Autodesk Fusion 360 part; units mm, degrees
(part 2 of 3)
  line L236 (-80.5456, -102.6502) -> (-76.5456, -102.6502)
  arc A232 (-58.9345, -105.6502) -> (-61.9345, -102.6502) centre (-61.9345, -105.6502) ccw
  line L237 (-58.9345, -105.6502) -> (-58.9345, -109.6502)
  arc A233 (-61.9345, -112.6502) -> (-58.9345, -109.6502) centre (-61.9345, -109.6502) ccw
  line L238 (-61.9345, -112.6502) -> (-65.9345, -112.6502)
  arc A234 (-68.9345, -109.6502) -> (-65.9345, -112.6502) centre (-65.9345, -109.6502) ccw
  line L239 (-68.9345, -109.6502) -> (-68.9345, -105.6502)
  arc A235 (-65.9345, -102.6502) -> (-68.9345, -105.6502) centre (-65.9345, -105.6502) ccw
  line L240 (-65.9345, -102.6502) -> (-61.9345, -102.6502)
  arc A236 (-44.3234, -105.6502) -> (-47.3234, -102.6502) centre (-47.3234, -105.6502) ccw
  line L241 (-44.3234, -105.6502) -> (-44.3234, -109.6502)
  arc A237 (-47.3234, -112.6502) -> (-44.3234, -109.6502) centre (-47.3234, -109.6502) ccw
  line L242 (-47.3234, -112.6502) -> (-51.3234, -112.6502)
  arc A238 (-54.3234, -109.6502) -> (-51.3234, -112.6502) centre (-51.3234, -109.6502) ccw
  line L243 (-54.3234, -109.6502) -> (-54.3234, -105.6502)
  arc A239 (-51.3234, -102.6502) -> (-54.3234, -105.6502) centre (-51.3234, -105.6502) ccw
  line L244 (-51.3234, -102.6502) -> (-47.3234, -102.6502)
  arc A240 (-29.7123, -105.6502) -> (-32.7123, -102.6502) centre (-32.7123, -105.6502) ccw
  line L245 (-29.7123, -105.6502) -> (-29.7123, -109.6502)
  arc A241 (-32.7123, -112.6502) -> (-29.7123, -109.6502) centre (-32.7123, -109.6502) ccw
  line L246 (-32.7123, -112.6502) -> (-36.7123, -112.6502)
  arc A242 (-39.7123, -109.6502) -> (-36.7123, -112.6502) centre (-36.7123, -109.6502) ccw
  line L247 (-39.7123, -109.6502) -> (-39.7123, -105.6502)
  arc A243 (-36.7123, -102.6502) -> (-39.7123, -105.6502) centre (-36.7123, -105.6502) ccw
  line L248 (-36.7123, -102.6502) -> (-32.7123, -102.6502)
  arc A244 (-161.2123, -120.2613) -> (-164.2123, -117.2613) centre (-164.2123, -120.2613) ccw
  line L249 (-161.2123, -120.2613) -> (-161.2123, -124.2613)
  arc A245 (-164.2123, -127.2613) -> (-161.2123, -124.2613) centre (-164.2123, -124.2613) ccw
  line L250 (-164.2123, -127.2613) -> (-168.2123, -127.2613)
  arc A246 (-171.2123, -124.2613) -> (-168.2123, -127.2613) centre (-168.2123, -124.2613) ccw
  line L251 (-171.2123, -124.2613) -> (-171.2123, -120.2613)
  arc A247 (-168.2123, -117.2613) -> (-171.2123, -120.2613) centre (-168.2123, -120.2613) ccw
  line L252 (-168.2123, -117.2613) -> (-164.2123, -117.2613)
  arc A248 (-146.6011, -120.2613) -> (-149.6011, -117.2613) centre (-149.6011, -120.2613) ccw
  line L253 (-146.6011, -120.2613) -> (-146.6011, -124.2613)
  arc A249 (-149.6011, -127.2613) -> (-146.6011, -124.2613) centre (-149.6011, -124.2613) ccw
  line L254 (-149.6011, -127.2613) -> (-153.6011, -127.2613)
  arc A250 (-156.6011, -124.2613) -> (-153.6011, -127.2613) centre (-153.6011, -124.2613) ccw
  line L255 (-156.6011, -124.2613) -> (-156.6011, -120.2613)
  arc A251 (-153.6011, -117.2613) -> (-156.6011, -120.2613) centre (-153.6011, -120.2613) ccw
  line L256 (-153.6011, -117.2613) -> (-149.6011, -117.2613)
  arc A252 (-131.99, -120.2613) -> (-134.99, -117.2613) centre (-134.99, -120.2613) ccw
  line L257 (-131.99, -120.2613) -> (-131.99, -124.2613)
  arc A253 (-134.99, -127.2613) -> (-131.99, -124.2613) centre (-134.99, -124.2613) ccw
  line L258 (-134.99, -127.2613) -> (-138.99, -127.2613)
  arc A254 (-141.99, -124.2613) -> (-138.99, -127.2613) centre (-138.99, -124.2613) ccw
  line L259 (-141.99, -124.2613) -> (-141.99, -120.2613)
  arc A255 (-138.99, -117.2613) -> (-141.99, -120.2613) centre (-138.99, -120.2613) ccw
  line L260 (-138.99, -117.2613) -> (-134.99, -117.2613)
  arc A256 (-117.3789, -120.2613) -> (-120.3789, -117.2613) centre (-120.3789, -120.2613) ccw
  line L261 (-117.3789, -120.2613) -> (-117.3789, -124.2613)
  arc A257 (-120.3789, -127.2613) -> (-117.3789, -124.2613) centre (-120.3789, -124.2613) ccw
  line L262 (-120.3789, -127.2613) -> (-124.3789, -127.2613)
  arc A258 (-127.3789, -124.2613) -> (-124.3789, -127.2613) centre (-124.3789, -124.2613) ccw
  line L263 (-127.3789, -124.2613) -> (-127.3789, -120.2613)
  arc A259 (-124.3789, -117.2613) -> (-127.3789, -120.2613) centre (-124.3789, -120.2613) ccw
  line L264 (-124.3789, -117.2613) -> (-120.3789, -117.2613)
  arc A260 (-102.7678, -120.2613) -> (-105.7678, -117.2613) centre (-105.7678, -120.2613) ccw
  line L265 (-102.7678, -120.2613) -> (-102.7678, -124.2613)
  arc A261 (-105.7678, -127.2613) -> (-102.7678, -124.2613) centre (-105.7678, -124.2613) ccw
  line L266 (-105.7678, -127.2613) -> (-109.7678, -127.2613)
  arc A262 (-112.7678, -124.2613) -> (-109.7678, -127.2613) centre (-109.7678, -124.2613) ccw
  line L267 (-112.7678, -124.2613) -> (-112.7678, -120.2613)
  arc A263 (-109.7678, -117.2613) -> (-112.7678, -120.2613) centre (-109.7678, -120.2613) ccw
  line L268 (-109.7678, -117.2613) -> (-105.7678, -117.2613)
  arc A264 (-88.1567, -120.2613) -> (-91.1567, -117.2613) centre (-91.1567, -120.2613) ccw
  line L269 (-88.1567, -120.2613) -> (-88.1567, -124.2613)
  arc A265 (-91.1567, -127.2613) -> (-88.1567, -124.2613) centre (-91.1567, -124.2613) ccw
  line L270 (-91.1567, -127.2613) -> (-95.1567, -127.2613)
  arc A266 (-98.1567, -124.2613) -> (-95.1567, -127.2613) centre (-95.1567, -124.2613) ccw
  line L271 (-98.1567, -124.2613) -> (-98.1567, -120.2613)
  arc A267 (-95.1567, -117.2613) -> (-98.1567, -120.2613) centre (-95.1567, -120.2613) ccw
  line L272 (-95.1567, -117.2613) -> (-91.1567, -117.2613)
  arc A268 (-73.5456, -120.2613) -> (-76.5456, -117.2613) centre (-76.5456, -120.2613) ccw
  line L273 (-73.5456, -120.2613) -> (-73.5456, -124.2613)
  arc A269 (-76.5456, -127.2613) -> (-73.5456, -124.2613) centre (-76.5456, -124.2613) ccw
  line L274 (-76.5456, -127.2613) -> (-80.5456, -127.2613)
  arc A270 (-83.5456, -124.2613) -> (-80.5456, -127.2613) centre (-80.5456, -124.2613) ccw
  line L275 (-83.5456, -124.2613) -> (-83.5456, -120.2613)
  arc A271 (-80.5456, -117.2613) -> (-83.5456, -120.2613) centre (-80.5456, -120.2613) ccw
  line L276 (-80.5456, -117.2613) -> (-76.5456, -117.2613)
  arc A272 (-58.9345, -120.2613) -> (-61.9345, -117.2613) centre (-61.9345, -120.2613) ccw
  line L277 (-58.9345, -120.2613) -> (-58.9345, -124.2613)
  arc A273 (-61.9345, -127.2613) -> (-58.9345, -124.2613) centre (-61.9345, -124.2613) ccw
  line L278 (-61.9345, -127.2613) -> (-65.9345, -127.2613)
  arc A274 (-68.9345, -124.2613) -> (-65.9345, -127.2613) centre (-65.9345, -124.2613) ccw
  line L279 (-68.9345, -124.2613) -> (-68.9345, -120.2613)
  arc A275 (-65.9345, -117.2613) -> (-68.9345, -120.2613) centre (-65.9345, -120.2613) ccw
  line L280 (-65.9345, -117.2613) -> (-61.9345, -117.2613)
  arc A276 (-44.3234, -120.2613) -> (-47.3234, -117.2613) centre (-47.3234, -120.2613) ccw
  line L281 (-44.3234, -120.2613) -> (-44.3234, -124.2613)
  arc A277 (-47.3234, -127.2613) -> (-44.3234, -124.2613) centre (-47.3234, -124.2613) ccw
  line L282 (-47.3234, -127.2613) -> (-51.3234, -127.2613)
  arc A278 (-54.3234, -124.2613) -> (-51.3234, -127.2613) centre (-51.3234, -124.2613) ccw
  line L283 (-54.3234, -124.2613) -> (-54.3234, -120.2613)
  arc A279 (-51.3234, -117.2613) -> (-54.3234, -120.2613) centre (-51.3234, -120.2613) ccw
  line L284 (-51.3234, -117.2613) -> (-47.3234, -117.2613)
  arc A280 (-29.7123, -120.2613) -> (-32.7123, -117.2613) centre (-32.7123, -120.2613) ccw
  line L285 (-29.7123, -120.2613) -> (-29.7123, -124.2613)
  arc A281 (-32.7123, -127.2613) -> (-29.7123, -124.2613) centre (-32.7123, -124.2613) ccw
  line L286 (-32.7123, -127.2613) -> (-36.7123, -127.2613)
  arc A282 (-39.7123, -124.2613) -> (-36.7123, -127.2613) centre (-36.7123, -124.2613) ccw
  line L287 (-39.7123, -124.2613) -> (-39.7123, -120.2613)
  arc A283 (-36.7123, -117.2613) -> (-39.7123, -120.2613) centre (-36.7123, -120.2613) ccw
  line L288 (-36.7123, -117.2613) -> (-32.7123, -117.2613)
  arc A284 (-161.2123, -134.8724) -> (-164.2123, -131.8724) centre (-164.2123, -134.8724) ccw
  line L289 (-161.2123, -134.8724) -> (-161.2123, -138.8724)
  arc A285 (-164.2123, -141.8724) -> (-161.2123, -138.8724) centre (-164.2123, -138.8724) ccw
  line L290 (-164.2123, -141.8724) -> (-168.2123, -141.8724)
  arc A286 (-171.2123, -138.8724) -> (-168.2123, -141.8724) centre (-168.2123, -138.8724) ccw
  line L291 (-171.2123, -138.8724) -> (-171.2123, -134.8724)
  arc A287 (-168.2123, -131.8724) -> (-171.2123, -134.8724) centre (-168.2123, -134.8724) ccw
  line L292 (-168.2123, -131.8724) -> (-164.2123, -131.8724)
  arc A288 (-146.6011, -134.8724) -> (-149.6011, -131.8724) centre (-149.6011, -134.8724) ccw
  line L293 (-146.6011, -134.8724) -> (-146.6011, -138.8724)
  arc A289 (-149.6011, -141.8724) -> (-146.6011, -138.8724) centre (-149.6011, -138.8724) ccw
  line L294 (-149.6011, -141.8724) -> (-153.6011, -141.8724)
  arc A290 (-156.6011, -138.8724) -> (-153.6011, -141.8724) centre (-153.6011, -138.8724) ccw
  line L295 (-156.6011, -138.8724) -> (-156.6011, -134.8724)
  arc A291 (-153.6011, -131.8724) -> (-156.6011, -134.8724) centre (-153.6011, -134.8724) ccw
  line L296 (-153.6011, -131.8724) -> (-149.6011, -131.8724)
  arc A292 (-131.99, -134.8724) -> (-134.99, -131.8724) centre (-134.99, -134.8724) ccw
  line L297 (-131.99, -134.8724) -> (-131.99, -138.8724)
  arc A293 (-134.99, -141.8724) -> (-131.99, -138.8724) centre (-134.99, -138.8724) ccw
  line L298 (-134.99, -141.8724) -> (-138.99, -141.8724)
  arc A294 (-141.99, -138.8724) -> (-138.99, -141.8724) centre (-138.99, -138.8724) ccw
  line L299 (-141.99, -138.8724) -> (-141.99, -134.8724)
  arc A295 (-138.99, -131.8724) -> (-141.99, -134.8724) centre (-138.99, -134.8724) ccw
  line L300 (-138.99, -131.8724) -> (-134.99, -131.8724)
  arc A296 (-117.3789, -134.8724) -> (-120.3789, -131.8724) centre (-120.3789, -134.8724) ccw
  line L301 (-117.3789, -134.8724) -> (-117.3789, -138.8724)
  arc A297 (-120.3789, -141.8724) -> (-117.3789, -138.8724) centre (-120.3789, -138.8724) ccw
  line L302 (-120.3789, -141.8724) -> (-124.3789, -141.8724)
  arc A298 (-127.3789, -138.8724) -> (-124.3789, -141.8724) centre (-124.3789, -138.8724) ccw
  line L303 (-127.3789, -138.8724) -> (-127.3789, -134.8724)
  arc A299 (-124.3789, -131.8724) -> (-127.3789, -134.8724) centre (-124.3789, -134.8724) ccw
  line L304 (-124.3789, -131.8724) -> (-120.3789, -131.8724)
  arc A300 (-102.7678, -134.8724) -> (-105.7678, -131.8724) centre (-105.7678, -134.8724) ccw
  line L305 (-102.7678, -134.8724) -> (-102.7678, -138.8724)
  arc A301 (-105.7678, -141.8724) -> (-102.7678, -138.8724) centre (-105.7678, -138.8724) ccw
  line L306 (-105.7678, -141.8724) -> (-109.7678, -141.8724)
  arc A302 (-112.7678, -138.8724) -> (-109.7678, -141.8724) centre (-109.7678, -138.8724) ccw
  line L307 (-112.7678, -138.8724) -> (-112.7678, -134.8724)
  arc A303 (-109.7678, -131.8724) -> (-112.7678, -134.8724) centre (-109.7678, -134.8724) ccw
  line L308 (-109.7678, -131.8724) -> (-105.7678, -131.8724)
  arc A304 (-88.1567, -134.8724) -> (-91.1567, -131.8724) centre (-91.1567, -134.8724) ccw
  line L309 (-88.1567, -134.8724) -> (-88.1567, -138.8724)
  arc A305 (-91.1567, -141.8724) -> (-88.1567, -138.8724) centre (-91.1567, -138.8724) ccw
  line L310 (-91.1567, -141.8724) -> (-95.1567, -141.8724)
  arc A306 (-98.1567, -138.8724) -> (-95.1567, -141.8724) centre (-95.1567, -138.8724) ccw
  line L311 (-98.1567, -138.8724) -> (-98.1567, -134.8724)
  arc A307 (-95.1567, -131.8724) -> (-98.1567, -134.8724) centre (-95.1567, -134.8724) ccw
  line L312 (-95.1567, -131.8724) -> (-91.1567, -131.8724)
  arc A308 (-73.5456, -134.8724) -> (-76.5456, -131.8724) centre (-76.5456, -134.8724) ccw
  line L313 (-73.5456, -134.8724) -> (-73.5456, -138.8724)
  arc A309 (-76.5456, -141.8724) -> (-73.5456, -138.8724) centre (-76.5456, -138.8724) ccw
  line L314 (-76.5456, -141.8724) -> (-80.5456, -141.8724)
  arc A310 (-83.5456, -138.8724) -> (-80.5456, -141.8724) centre (-80.5456, -138.8724) ccw
  line L315 (-83.5456, -138.8724) -> (-83.5456, -134.8724)
  arc A311 (-80.5456, -131.8724) -> (-83.5456, -134.8724) centre (-80.5456, -134.8724) ccw
  line L316 (-80.5456, -131.8724) -> (-76.5456, -131.8724)
  arc A312 (-58.9345, -134.8724) -> (-61.9345, -131.8724) centre (-61.9345, -134.8724) ccw
  line L317 (-58.9345, -134.8724) -> (-58.9345, -138.8724)
  arc A313 (-61.9345, -141.8724) -> (-58.9345, -138.8724) centre (-61.9345, -138.8724) ccw
  line L318 (-61.9345, -141.8724) -> (-65.9345, -141.8724)
  arc A314 (-68.9345, -138.8724) -> (-65.9345, -141.8724) centre (-65.9345, -138.8724) ccw
  line L319 (-68.9345, -138.8724) -> (-68.9345, -134.8724)
  arc A315 (-65.9345, -131.8724) -> (-68.9345, -134.8724) centre (-65.9345, -134.8724) ccw
  line L320 (-65.9345, -131.8724) -> (-61.9345, -131.8724)
  arc A316 (-44.3234, -134.8724) -> (-47.3234, -131.8724) centre (-47.3234, -134.8724) ccw
  line L321 (-44.3234, -134.8724) -> (-44.3234, -138.8724)
  arc A317 (-47.3234, -141.8724) -> (-44.3234, -138.8724) centre (-47.3234, -138.8724) ccw
  line L322 (-47.3234, -141.8724) -> (-51.3234, -141.8724)
  arc A318 (-54.3234, -138.8724) -> (-51.3234, -141.8724) centre (-51.3234, -138.8724) ccw
  line L323 (-54.3234, -138.8724) -> (-54.3234, -134.8724)
  arc A319 (-51.3234, -131.8724) -> (-54.3234, -134.8724) centre (-51.3234, -134.8724) ccw
  line L324 (-51.3234, -131.8724) -> (-47.3234, -131.8724)
  arc A320 (-29.7123, -134.8724) -> (-32.7123, -131.8724) centre (-32.7123, -134.8724) ccw
  line L325 (-29.7123, -134.8724) -> (-29.7123, -138.8724)
  arc A321 (-32.7123, -141.8724) -> (-29.7123, -138.8724) centre (-32.7123, -138.8724) ccw
  line L326 (-32.7123, -141.8724) -> (-36.7123, -141.8724)
  arc A322 (-39.7123, -138.8724) -> (-36.7123, -141.8724) centre (-36.7123, -138.8724) ccw
  line L327 (-39.7123, -138.8724) -> (-39.7123, -134.8724)
  arc A323 (-36.7123, -131.8724) -> (-39.7123, -134.8724) centre (-36.7123, -134.8724) ccw
  line L328 (-36.7123, -131.8724) -> (-32.7123, -131.8724)
  arc A324 (-161.2123, -149.4835) -> (-164.2123, -146.4835) centre (-164.2123, -149.4835) ccw
  line L329 (-161.2123, -149.4835) -> (-161.2123, -153.4835)
  arc A325 (-164.2123, -156.4835) -> (-161.2123, -153.4835) centre (-164.2123, -153.4835) ccw
  line L330 (-164.2123, -156.4835) -> (-168.2123, -156.4835)
  arc A326 (-171.2123, -153.4835) -> (-168.2123, -156.4835) centre (-168.2123, -153.4835) ccw
  line L331 (-171.2123, -153.4835) -> (-171.2123, -149.4835)
  arc A327 (-168.2123, -146.4835) -> (-171.2123, -149.4835) centre (-168.2123, -149.4835) ccw
  line L332 (-168.2123, -146.4835) -> (-164.2123, -146.4835)
  arc A328 (-146.6011, -149.4835) -> (-149.6011, -146.4835) centre (-149.6011, -149.4835) ccw
  line L333 (-146.6011, -149.4835) -> (-146.6011, -153.4835)
  arc A329 (-149.6011, -156.4835) -> (-146.6011, -153.4835) centre (-149.6011, -153.4835) ccw
  line L334 (-149.6011, -156.4835) -> (-153.6011, -156.4835)
  arc A330 (-156.6011, -153.4835) -> (-153.6011, -156.4835) centre (-153.6011, -153.4835) ccw
  line L335 (-156.6011, -153.4835) -> (-156.6011, -149.4835)
  arc A331 (-153.6011, -146.4835) -> (-156.6011, -149.4835) centre (-153.6011, -149.4835) ccw
  line L336 (-153.6011, -146.4835) -> (-149.6011, -146.4835)
  arc A332 (-131.99, -149.4835) -> (-134.99, -146.4835) centre (-134.99, -149.4835) ccw
  line L337 (-131.99, -149.4835) -> (-131.99, -153.4835)
  arc A333 (-134.99, -156.4835) -> (-131.99, -153.4835) centre (-134.99, -153.4835) ccw
  line L338 (-134.99, -156.4835) -> (-138.99, -156.4835)
  arc A334 (-141.99, -153.4835) -> (-138.99, -156.4835) centre (-138.99, -153.4835) ccw
  line L339 (-141.99, -153.4835) -> (-141.99, -149.4835)
  arc A335 (-138.99, -146.4835) -> (-141.99, -149.4835) centre (-138.99, -149.4835) ccw
  line L340 (-138.99, -146.4835) -> (-134.99, -146.4835)
  arc A336 (-117.3789, -149.4835) -> (-120.3789, -146.4835) centre (-120.3789, -149.4835) ccw
  line L341 (-117.3789, -149.4835) -> (-117.3789, -153.4835)
  arc A337 (-120.3789, -156.4835) -> (-117.3789, -153.4835) centre (-120.3789, -153.4835) ccw
  line L342 (-120.3789, -156.4835) -> (-124.3789, -156.4835)
  arc A338 (-127.3789, -153.4835) -> (-124.3789, -156.4835) centre (-124.3789, -153.4835) ccw
  line L343 (-127.3789, -153.4835) -> (-127.3789, -149.4835)
  arc A339 (-124.3789, -146.4835) -> (-127.3789, -149.4835) centre (-124.3789, -149.4835) ccw
  line L344 (-124.3789, -146.4835) -> (-120.3789, -146.4835)
  arc A340 (-102.7678, -149.4835) -> (-105.7678, -146.4835) centre (-105.7678, -149.4835) ccw
  line L345 (-102.7678, -149.4835) -> (-102.7678, -153.4835)
  arc A341 (-105.7678, -156.4835) -> (-102.7678, -153.4835) centre (-105.7678, -153.4835) ccw
  line L346 (-105.7678, -156.4835) -> (-109.7678, -156.4835)
  arc A342 (-112.7678, -153.4835) -> (-109.7678, -156.4835) centre (-109.7678, -153.4835) ccw
  line L347 (-112.7678, -153.4835) -> (-112.7678, -149.4835)
  arc A343 (-109.7678, -146.4835) -> (-112.7678, -149.4835) centre (-109.7678, -149.4835) ccw
  line L348 (-109.7678, -146.4835) -> (-105.7678, -146.4835)
  arc A344 (-88.1567, -149.4835) -> (-91.1567, -146.4835) centre (-91.1567, -149.4835) ccw
  line L349 (-88.1567, -149.4835) -> (-88.1567, -153.4835)
  arc A345 (-91.1567, -156.4835) -> (-88.1567, -153.4835) centre (-91.1567, -153.4835) ccw
  line L350 (-91.1567, -156.4835) -> (-95.1567, -156.4835)
  arc A346 (-98.1567, -153.4835) -> (-95.1567, -156.4835) centre (-95.1567, -153.4835) ccw
  line L351 (-98.1567, -153.4835) -> (-98.1567, -149.4835)
  arc A347 (-95.1567, -146.4835) -> (-98.1567, -149.4835) centre (-95.1567, -149.4835) ccw
  line L352 (-95.1567, -146.4835) -> (-91.1567, -146.4835)
  arc A348 (-73.5456, -149.4835) -> (-76.5456, -146.4835) centre (-76.5456, -149.4835) ccw
  line L353 (-73.5456, -149.4835) -> (-73.5456, -153.4835)
  arc A349 (-76.5456, -156.4835) -> (-73.5456, -153.4835) centre (-76.5456, -153.4835) ccw
  line L354 (-76.5456, -156.4835) -> (-80.5456, -156.4835)
  arc A350 (-83.5456, -153.4835) -> (-80.5456, -156.4835) centre (-80.5456, -153.4835) ccw
  line L355 (-83.5456, -153.4835) -> (-83.5456, -149.4835)
  arc A351 (-80.5456, -146.4835) -> (-83.5456, -149.4835) centre (-80.5456, -149.4835) ccw
  line L356 (-80.5456, -146.4835) -> (-76.5456, -146.4835)
  arc A352 (-58.9345, -149.4835) -> (-61.9345, -146.4835) centre (-61.9345, -149.4835) ccw
  line L357 (-58.9345, -149.4835) -> (-58.9345, -153.4835)
  arc A353 (-61.9345, -156.4835) -> (-58.9345, -153.4835) centre (-61.9345, -153.4835) ccw
  line L358 (-61.9345, -156.4835) -> (-65.9345, -156.4835)
  arc A354 (-68.9345, -153.4835) -> (-65.9345, -156.4835) centre (-65.9345, -153.4835) ccw
  line L359 (-68.9345, -153.4835) -> (-68.9345, -149.4835)
  arc A355 (-65.9345, -146.4835) -> (-68.9345, -149.4835) centre (-65.9345, -149.4835) ccw
  line L360 (-65.9345, -146.4835) -> (-61.9345, -146.4835)
  arc A356 (-44.3234, -149.4835) -> (-47.3234, -146.4835) centre (-47.3234, -149.4835) ccw
  line L361 (-44.3234, -149.4835) -> (-44.3234, -153.4835)
  arc A357 (-47.3234, -156.4835) -> (-44.3234, -153.4835) centre (-47.3234, -153.4835) ccw
  line L362 (-47.3234, -156.4835) -> (-51.3234, -156.4835)
  arc A358 (-54.3234, -153.4835) -> (-51.3234, -156.4835) centre (-51.3234, -153.4835) ccw
  line L363 (-54.3234, -153.4835) -> (-54.3234, -149.4835)
  arc A359 (-51.3234, -146.4835) -> (-54.3234, -149.4835) centre (-51.3234, -149.4835) ccw
  line L364 (-51.3234, -146.4835) -> (-47.3234, -146.4835)
  arc A360 (-29.7123, -149.4835) -> (-32.7123, -146.4835) centre (-32.7123, -149.4835) ccw
  line L365 (-29.7123, -149.4835) -> (-29.7123, -153.4835)
  arc A361 (-32.7123, -156.4835) -> (-29.7123, -153.4835) centre (-32.7123, -153.4835) ccw
  line L366 (-32.7123, -156.4835) -> (-36.7123, -156.4835)
  arc A362 (-39.7123, -153.4835) -> (-36.7123, -156.4835) centre (-36.7123, -153.4835) ccw
  line L367 (-39.7123, -153.4835) -> (-39.7123, -149.4835)
  arc A363 (-36.7123, -146.4835) -> (-39.7123, -149.4835) centre (-36.7123, -149.4835) ccw
  line L368 (-36.7123, -146.4835) -> (-32.7123, -146.4835)
  arc A364 (-161.2123, -164.0946) -> (-164.2123, -161.0946) centre (-164.2123, -164.0946) ccw
  line L369 (-161.2123, -164.0946) -> (-161.2123, -168.0946)
  arc A365 (-164.2123, -171.0946) -> (-161.2123, -168.0946) centre (-164.2123, -168.0946) ccw
  line L370 (-164.2123, -171.0946) -> (-168.2123, -171.0946)
  arc A366 (-171.2123, -168.0946) -> (-168.2123, -171.0946) centre (-168.2123, -168.0946) ccw
  line L371 (-171.2123, -168.0946) -> (-171.2123, -164.0946)
  arc A367 (-168.2123, -161.0946) -> (-171.2123, -164.0946) centre (-168.2123, -164.0946) ccw
  line L372 (-168.2123, -161.0946) -> (-164.2123, -161.0946)
  arc A368 (-146.6011, -164.0946) -> (-149.6011, -161.0946) centre (-149.6011, -164.0946) ccw
  line L373 (-146.6011, -164.0946) -> (-146.6011, -168.0946)
  arc A369 (-149.6011, -171.0946) -> (-146.6011, -168.0946) centre (-149.6011, -168.0946) ccw
  line L374 (-149.6011, -171.0946) -> (-153.6011, -171.0946)
  arc A370 (-156.6011, -168.0946) -> (-153.6011, -171.0946) centre (-153.6011, -168.0946) ccw
  line L375 (-156.6011, -168.0946) -> (-156.6011, -164.0946)
  arc A371 (-153.6011, -161.0946) -> (-156.6011, -164.0946) centre (-153.6011, -164.0946) ccw
  line L376 (-153.6011, -161.0946) -> (-149.6011, -161.0946)
  arc A372 (-131.99, -164.0946) -> (-134.99, -161.0946) centre (-134.99, -164.0946) ccw
  line L377 (-131.99, -164.0946) -> (-131.99, -168.0946)
  arc A373 (-134.99, -171.0946) -> (-131.99, -168.0946) centre (-134.99, -168.0946) ccw
  line L378 (-134.99, -171.0946) -> (-138.99, -171.0946)
  arc A374 (-141.99, -168.0946) -> (-138.99, -171.0946) centre (-138.99, -168.0946) ccw
  line L379 (-141.99, -168.0946) -> (-141.99, -164.0946)
  arc A375 (-138.99, -161.0946) -> (-141.99, -164.0946) centre (-138.99, -164.0946) ccw
  line L380 (-138.99, -161.0946) -> (-134.99, -161.0946)
  arc A376 (-117.3789, -164.0946) -> (-120.3789, -161.0946) centre (-120.3789, -164.0946) ccw
  line L381 (-117.3789, -164.0946) -> (-117.3789, -168.0946)
  arc A377 (-120.3789, -171.0946) -> (-117.3789, -168.0946) centre (-120.3789, -168.0946) ccw
  line L382 (-120.3789, -171.0946) -> (-124.3789, -171.0946)
  arc A378 (-127.3789, -168.0946) -> (-124.3789, -171.0946) centre (-124.3789, -168.0946) ccw
  line L383 (-127.3789, -168.0946) -> (-127.3789, -164.0946)
  arc A379 (-124.3789, -161.0946) -> (-127.3789, -164.0946) centre (-124.3789, -164.0946) ccw
  line L384 (-124.3789, -161.0946) -> (-120.3789, -161.0946)
  arc A380 (-102.7678, -164.0946) -> (-105.7678, -161.0946) centre (-105.7678, -164.0946) ccw
  line L385 (-102.7678, -164.0946) -> (-102.7678, -168.0946)
  arc A381 (-105.7678, -171.0946) -> (-102.7678, -168.0946) centre (-105.7678, -168.0946) ccw
  line L386 (-105.7678, -171.0946) -> (-109.7678, -171.0946)
  arc A382 (-112.7678, -168.0946) -> (-109.7678, -171.0946) centre (-109.7678, -168.0946) ccw
  line L387 (-112.7678, -168.0946) -> (-112.7678, -164.0946)
  arc A383 (-109.7678, -161.0946) -> (-112.7678, -164.0946) centre (-109.7678, -164.0946) ccw
  line L388 (-109.7678, -161.0946) -> (-105.7678, -161.0946)
  arc A384 (-88.1567, -164.0946) -> (-91.1567, -161.0946) centre (-91.1567, -164.0946) ccw
  line L389 (-88.1567, -164.0946) -> (-88.1567, -168.0946)
  arc A385 (-91.1567, -171.0946) -> (-88.1567, -168.0946) centre (-91.1567, -168.0946) ccw
  line L390 (-91.1567, -171.0946) -> (-95.1567, -171.0946)
  arc A386 (-98.1567, -168.0946) -> (-95.1567, -171.0946) centre (-95.1567, -168.0946) ccw
  line L391 (-98.1567, -168.0946) -> (-98.1567, -164.0946)
  arc A387 (-95.1567, -161.0946) -> (-98.1567, -164.0946) centre (-95.1567, -164.0946) ccw
  line L392 (-95.1567, -161.0946) -> (-91.1567, -161.0946)
  arc A388 (-73.5456, -164.0946) -> (-76.5456, -161.0946) centre (-76.5456, -164.0946) ccw
  line L393 (-73.5456, -164.0946) -> (-73.5456, -168.0946)
  arc A389 (-76.5456, -171.0946) -> (-73.5456, -168.0946) centre (-76.5456, -168.0946) ccw
  line L394 (-76.5456, -171.0946) -> (-80.5456, -171.0946)
  arc A390 (-83.5456, -168.0946) -> (-80.5456, -171.0946) centre (-80.5456, -168.0946) ccw
  line L395 (-83.5456, -168.0946) -> (-83.5456, -164.0946)
  arc A391 (-80.5456, -161.0946) -> (-83.5456, -164.0946) centre (-80.5456, -164.0946) ccw
  line L396 (-80.5456, -161.0946) -> (-76.5456, -161.0946)
  arc A392 (-58.9345, -164.0946) -> (-61.9345, -161.0946) centre (-61.9345, -164.0946) ccw
  line L397 (-58.9345, -164.0946) -> (-58.9345, -168.0946)
  arc A393 (-61.9345, -171.0946) -> (-58.9345, -168.0946) centre (-61.9345, -168.0946) ccw
  line L398 (-61.9345, -171.0946) -> (-65.9345, -171.0946)
  arc A394 (-68.9345, -168.0946) -> (-65.9345, -171.0946) centre (-65.9345, -168.0946) ccw
  line L399 (-68.9345, -168.0946) -> (-68.9345, -164.0946)
  arc A395 (-65.9345, -161.0946) -> (-68.9345, -164.0946) centre (-65.9345, -164.0946) ccw
  line L400 (-65.9345, -161.0946) -> (-61.9345, -161.0946)
  arc A396 (-44.3234, -164.0946) -> (-47.3234, -161.0946) centre (-47.3234, -164.0946) ccw
  line L401 (-44.3234, -164.0946) -> (-44.3234, -168.0946)
  arc A397 (-47.3234, -171.0946) -> (-44.3234, -168.0946) centre (-47.3234, -168.0946) ccw
  line L402 (-47.3234, -171.0946) -> (-51.3234, -171.0946)
  arc A398 (-54.3234, -168.0946) -> (-51.3234, -171.0946) centre (-51.3234, -168.0946) ccw
  line L403 (-54.3234, -168.0946) -> (-54.3234, -164.0946)
  arc A399 (-51.3234, -161.0946) -> (-54.3234, -164.0946) centre (-51.3234, -164.0946) ccw
  line L404 (-51.3234, -161.0946) -> (-47.3234, -161.0946)
  arc A400 (-29.7123, -164.0946) -> (-32.7123, -161.0946) centre (-32.7123, -164.0946) ccw
  line L405 (-29.7123, -164.0946) -> (-29.7123, -168.0946)
  arc A401 (-32.7123, -171.0946) -> (-29.7123, -168.0946) centre (-32.7123, -168.0946) ccw
  line L406 (-32.7123, -171.0946) -> (-36.7123, -171.0946)
  arc A402 (-39.7123, -168.0946) -> (-36.7123, -171.0946) centre (-36.7123, -168.0946) ccw
  line L407 (-39.7123, -168.0946) -> (-39.7123, -164.0946)
  arc A403 (-36.7123, -161.0946) -> (-39.7123, -164.0946) centre (-36.7123, -164.0946) ccw
  line L408 (-36.7123, -161.0946) -> (-32.7123, -161.0946)
  point P0 (-166.2123, -34.5946)
  dimension "d125" = 10
  dimension "d126" = 10
  dimension "d127" = 3
  dimension "d128" = 3
  dimension "d131" = 0
  dimension "d132" = 0
  dimension "d135" = 131.5
  dimension "d136" = -131.5
  constraint horizontal L7
  constraint perpendicular L7 L8
  constraint parallel L7 L9
  constraint parallel L8 L10
  constraint coincident L11 P0
  constraint coincident L12 P0
  constraint coincident P0 A0.centre
  constraint coincident L12.end L10
  constraint coincident L12.end L9
  constraint tangent L10 A4
  constraint tangent L9 A4
  constraint coincident L11.end L9
  constraint coincident L11.end L8
  constraint tangent L9 A5
  constraint tangent L8 A5
  constraint equal A4 A5
  constraint coincident L12.start L8
  constraint coincident L12.start L7
  constraint tangent L8 A6
  constraint tangent L7 A6
  constraint equal A4 A6
  constraint coincident L11.start L7
  constraint coincident L11.start L10
  constraint tangent L7 A7
  constraint tangent L10 A7
  measures "d125" distance of L11.end L12.end
  measures "d126" distance of L12.start L11.end
  measures "d127" radius of A4
  measures "d128" radius of A7
extrude "Extrude30" cut sketch "Sketch12" against normal blind 10 contours L7 L8 L9 L10 A4 A5 A6 A7 | A8 L13 A9 L14 A10 L15 A11 L16 | A12 L17 A13 L18 A14 L19 A15 L20 | A16 L21 A17 L22 A18 L23 A19 L24 | A20 L25 A21 L26 A22 L27 A23 L28 | A24 L29 A25 L30 A26 L31 A27 L32 | A28 L33 A29 L34 A30 L35 A31 L36 | A32 L37 A33 L38 A34 L39 A35 L40 | A36 L41 A37 L42 A38 L43 A39 L44 | A40 L45 A41 L46 A42 L47 A43 L48 | A44 L49 A45 L50 A46 L51 A47 L52 | A48 L53 A49 L54 A50 L55 A51 L56 | A52 L57 A53 L58 A54 L59 A55 L60 | A56 L61 A57 L62 A58 L63 A59 L64 | A60 L65 A61 L66 A62 L67 A63 L68 | A64 L69 A65 L70 A66 L71 A67 L72 | A68 L73 A69 L74 A70 L75 A71 L76 | A72 L77 A73 L78 A74 L79 A75 L80 | A76 L81 A77 L82 A78 L83 A79 L84 | A80 L85 A81 L86 A82 L87 A83 L88 | A84 L89 A85 L90 A86 L91 A87 L92 | A88 L93 A89 L94 A90 L95 A91 L96 | A92 L97 A93 L98 A94 L99 A95 L100 | A96 L101 A97 L102 A98 L103 A99 L104 | A100 L105 A101 L106 A102 L107 A103 L108 | A104 L109 A105 L110 A106 L111 A107 L112 | A108 L113 A109 L114 A110 L115 A111 L116 | A112 L117 A113 L118 A114 L119 A115 L120 | A116 L121 A117 L122 A118 L123 A119 L124 | A120 L125 A121 L126 A122 L127 A123 L128 | A124 L129 A125 L130 A126 L131 A127 L132 | A128 L133 A129 L134 A130 L135 A131 L136 | A132 L137 A133 L138 A134 L139 A135 L140 | A136 L141 A137 L142 A138 L143 A139 L144 | A140 L145 A141 L146 A142 L147 A143 L148 | A144 L149 A145 L150 A146 L151 A147 L152 | A148 L153 A149 L154 A150 L155 A151 L156 | A152 L157 A153 L158 A154 L159 A155 L160 | A156 L161 A157 L162 A158 L163 A159 L164 | A160 L165 A161 L166 A162 L167 A163 L168 | A164 L169 A165 L170 A166 L171 A167 L172 | A168 L173 A169 L174 A170 L175 A171 L176 | A172 L177 A173 L178 A174 L179 A175 L180 | A176 L181 A177 L182 A178 L183 A179 L184 | A180 L185 A181 L186 A182 L187 A183 L188 | A184 L189 A185 L190 A186 L191 A187 L192 | A188 L193 A189 L194 A190 L195 A191 L196 | A192 L197 A193 L198 A194 L199 A195 L200 | A196 L201 A197 L202 A198 L203 A199 L204 | A200 L205 A201 L206 A202 L207 A203 L208 | A204 L209 A205 L210 A206 L211 A207 L212 | A208 L213 A209 L214 A210 L215 A211 L216 | A212 L217 A213 L218 A214 L219 A215 L220 | A216 L221 A217 L222 A218 L223 A219 L224 | A220 L225 A221 L226 A222 L227 A223 L228 | A224 L229 A225 L230 A226 L231 A227 L232 | A228 L233 A229 L234 A230 L235 A231 L236 | A232 L237 A233 L238 A234 L239 A235 L240 | A236 L241 A237 L242 A238 L243 A239 L244 | A240 L245 A241 L246 A242 L247 A243 L248 | A244 L249 A245 L250 A246 L251 A247 L252 | A248 L253 A249 L254 A250 L255 A251 L256 | A252 L257 A253 L258 A254 L259 A255 L260 | A256 L261 A257 L262 A258 L263 A259 L264 | A260 L265 A261 L266 A262 L267 A263 L268 | A264 L269 A265 L270 A266 L271 A267 L272 | A268 L273 A269 L274 A270 L275 A271 L276 | A272 L277 A273 L278 A274 L279 A275 L280 | A276 L281 A277 L282 A278 L283 A279 L284 | A280 L285 A281 L286 A282 L287 A283 L288 | A284 L289 A285 L290 A286 L291 A287 L292 | A288 L293 A289 L294 A290 L295 A291 L296 | A292 L297 A293 L298 A294 L299 A295 L300 | A296 L301 A297 L302 A298 L303 A299 L304 | A300 L305 A301 L306 A302 L307 A303 L308 | A304 L309 A305 L310 A306 L311 A307 L312 | A308 L313 A309 L314 A310 L315 A311 L316 | A312 L317 A313 L318 A314 L319 A315 L320 | A316 L321 A317 L322 A318 L323 A319 L324 | A320 L325 A321 L326 A322 L327 A323 L328 | A324 L329 A325 L330 A326 L331 A327 L332 | A328 L333 A329 L334 A330 L335 A331 L336 | A332 L337 A333 L338 A334 L339 A335 L340 | A336 L341 A337 L342 A338 L343 A339 L344 | A340 L345 A341 L346 A342 L347 A343 L348 | A344 L349 A345 L350 A346 L351 A347 L352 | A348 L353 A349 L354 A350 L355 A351 L356 | A352 L357 A353 L358 A354 L359 A355 L360 | A356 L361 A357 L362 A358 L363 A359 L364 | A360 L365 A361 L366 A362 L367 A363 L368 | A364 L369 A365 L370 A366 L371 A367 L372 | A368 L373 A369 L374 A370 L375 A371 L376 | A372 L377 A373 L378 A374 L379 A375 L380 | A376 L381 A377 L382 A378 L383 A379 L384 | A380 L385 A381 L386 A382 L387 A383 L388 | A384 L389 A385 L390 A386 L391 A387 L392 | A388 L393 A389 L394 A390 L395 A391 L396 | A392 L397 A393 L398 A394 L399 A395 L400 | A396 L401 A397 L402 A398 L403 A399 L404 | A400 L405 A401 L406 A402 L407 A403 L408 bodies 11
sketch "Sketch13" plane through (0, 0, 2) normal (0, 0, 1) x (-1, 0, 0)
  line L0 (-149.6011, -83.428) -> (-153.6011, -83.428)
  arc A0 (-156.6011, -80.428) -> (-153.6011, -83.428) centre (-153.6011, -80.428) ccw
  line L1 (-156.6011, -80.428) -> (-156.6011, -76.428)
  arc A1 (-153.6011, -73.428) -> (-156.6011, -76.428) centre (-153.6011, -76.428) ccw
  line L2 (-153.6011, -73.428) -> (-149.6011, -73.428)
  arc A2 (-146.6011, -76.428) -> (-149.6011, -73.428) centre (-149.6011, -76.428) ccw
  line L3 (-146.6011, -76.428) -> (-146.6011, -80.428)
  arc A3 (-149.6011, -83.428) -> (-146.6011, -80.428) centre (-149.6011, -80.428) ccw
  line L4 (-32.7123, -141.8724) -> (-36.7123, -141.8724)
  arc A4 (-39.7123, -138.8724) -> (-36.7123, -141.8724) centre (-36.7123, -138.8724) ccw
  line L5 (-39.7123, -138.8724) -> (-39.7123, -134.8724)
  arc A5 (-36.7123, -131.8724) -> (-39.7123, -134.8724) centre (-36.7123, -134.8724) ccw
  line L6 (-36.7123, -131.8724) -> (-32.7123, -131.8724)
  arc A6 (-29.7123, -134.8724) -> (-32.7123, -131.8724) centre (-32.7123, -134.8724) ccw
  line L7 (-29.7123, -134.8724) -> (-29.7123, -138.8724)
  arc A7 (-32.7123, -141.8724) -> (-29.7123, -138.8724) centre (-32.7123, -138.8724) ccw
  line L8 (-76.5456, -156.4835) -> (-80.5456, -156.4835)
  arc A8 (-83.5456, -153.4835) -> (-80.5456, -156.4835) centre (-80.5456, -153.4835) ccw
  line L9 (-83.5456, -153.4835) -> (-83.5456, -149.4835)
  arc A9 (-80.5456, -146.4835) -> (-83.5456, -149.4835) centre (-80.5456, -149.4835) ccw
  line L10 (-80.5456, -146.4835) -> (-76.5456, -146.4835)
  arc A10 (-73.5456, -149.4835) -> (-76.5456, -146.4835) centre (-76.5456, -149.4835) ccw
  line L11 (-73.5456, -149.4835) -> (-73.5456, -153.4835)
  arc A11 (-76.5456, -156.4835) -> (-73.5456, -153.4835) centre (-76.5456, -153.4835) ccw
  line L12 (-120.3789, -54.2058) -> (-124.3789, -54.2058)
  arc A12 (-127.3789, -51.2058) -> (-124.3789, -54.2058) centre (-124.3789, -51.2058) ccw
  line L13 (-127.3789, -51.2058) -> (-127.3789, -47.2058)
  arc A13 (-124.3789, -44.2058) -> (-127.3789, -47.2058) centre (-124.3789, -47.2058) ccw
  line L14 (-124.3789, -44.2058) -> (-120.3789, -44.2058)
  arc A14 (-117.3789, -47.2058) -> (-120.3789, -44.2058) centre (-120.3789, -47.2058) ccw
  line L15 (-117.3789, -47.2058) -> (-117.3789, -51.2058)
  arc A15 (-120.3789, -54.2058) -> (-117.3789, -51.2058) centre (-120.3789, -51.2058) ccw
  line L16 (-120.3789, -98.0391) -> (-124.3789, -98.0391)
  arc A16 (-127.3789, -95.0391) -> (-124.3789, -98.0391) centre (-124.3789, -95.0391) ccw
  line L17 (-127.3789, -95.0391) -> (-127.3789, -91.0391)
  arc A17 (-124.3789, -88.0391) -> (-127.3789, -91.0391) centre (-124.3789, -91.0391) ccw
  line L18 (-124.3789, -88.0391) -> (-120.3789, -88.0391)
  arc A18 (-117.3789, -91.0391) -> (-120.3789, -88.0391) centre (-120.3789, -91.0391) ccw
  line L19 (-117.3789, -91.0391) -> (-117.3789, -95.0391)
  arc A19 (-120.3789, -98.0391) -> (-117.3789, -95.0391) centre (-120.3789, -95.0391) ccw
  line L20 (-105.7678, -127.2613) -> (-109.7678, -127.2613)
  arc A20 (-112.7678, -124.2613) -> (-109.7678, -127.2613) centre (-109.7678, -124.2613) ccw
  line L21 (-112.7678, -124.2613) -> (-112.7678, -120.2613)
  arc A21 (-109.7678, -117.2613) -> (-112.7678, -120.2613) centre (-109.7678, -120.2613) ccw
  line L22 (-109.7678, -117.2613) -> (-105.7678, -117.2613)
  arc A22 (-102.7678, -120.2613) -> (-105.7678, -117.2613) centre (-105.7678, -120.2613) ccw
  line L23 (-102.7678, -120.2613) -> (-102.7678, -124.2613)
  arc A23 (-105.7678, -127.2613) -> (-102.7678, -124.2613) centre (-105.7678, -124.2613) ccw
  line L24 (-134.99, -54.2058) -> (-138.99, -54.2058)
  arc A24 (-141.99, -51.2058) -> (-138.99, -54.2058) centre (-138.99, -51.2058) ccw
  line L25 (-141.99, -51.2058) -> (-141.99, -47.2058)
  arc A25 (-138.99, -44.2058) -> (-141.99, -47.2058) centre (-138.99, -47.2058) ccw
  line L26 (-138.99, -44.2058) -> (-134.99, -44.2058)
  arc A26 (-131.99, -47.2058) -> (-134.99, -44.2058) centre (-134.99, -47.2058) ccw
  line L27 (-131.99, -47.2058) -> (-131.99, -51.2058)
  arc A27 (-134.99, -54.2058) -> (-131.99, -51.2058) centre (-134.99, -51.2058) ccw
  line L28 (-134.99, -83.428) -> (-138.99, -83.428)
  arc A28 (-141.99, -80.428) -> (-138.99, -83.428) centre (-138.99, -80.428) ccw
  line L29 (-141.99, -80.428) -> (-141.99, -76.428)
  arc A29 (-138.99, -73.428) -> (-141.99, -76.428) centre (-138.99, -76.428) ccw
  line L30 (-138.99, -73.428) -> (-134.99, -73.428)
  arc A30 (-131.99, -76.428) -> (-134.99, -73.428) centre (-134.99, -76.428) ccw
  line L31 (-131.99, -76.428) -> (-131.99, -80.428)
  arc A31 (-134.99, -83.428) -> (-131.99, -80.428) centre (-134.99, -80.428) ccw
  line L32 (-134.99, -112.6502) -> (-138.99, -112.6502)
  arc A32 (-141.99, -109.6502) -> (-138.99, -112.6502) centre (-138.99, -109.6502) ccw
  line L33 (-141.99, -109.6502) -> (-141.99, -105.6502)
  arc A33 (-138.99, -102.6502) -> (-141.99, -105.6502) centre (-138.99, -105.6502) ccw
  line L34 (-138.99, -102.6502) -> (-134.99, -102.6502)
  arc A34 (-131.99, -105.6502) -> (-134.99, -102.6502) centre (-134.99, -105.6502) ccw
  line L35 (-131.99, -105.6502) -> (-131.99, -109.6502)
  arc A35 (-134.99, -112.6502) -> (-131.99, -109.6502) centre (-134.99, -109.6502) ccw
  line L36 (-105.7678, -98.0391) -> (-109.7678, -98.0391)
  arc A36 (-112.7678, -95.0391) -> (-109.7678, -98.0391) centre (-109.7678, -95.0391) ccw
  line L37 (-112.7678, -95.0391) -> (-112.7678, -91.0391)
  arc A37 (-109.7678, -88.0391) -> (-112.7678, -91.0391) centre (-109.7678, -91.0391) ccw
  line L38 (-109.7678, -88.0391) -> (-105.7678, -88.0391)
  arc A38 (-102.7678, -91.0391) -> (-105.7678, -88.0391) centre (-105.7678, -91.0391) ccw
  line L39 (-102.7678, -91.0391) -> (-102.7678, -95.0391)
  arc A39 (-105.7678, -98.0391) -> (-102.7678, -95.0391) centre (-105.7678, -95.0391) ccw
  line L40 (-120.3789, -83.428) -> (-124.3789, -83.428)
  arc A40 (-127.3789, -80.428) -> (-124.3789, -83.428) centre (-124.3789, -80.428) ccw
  line L41 (-127.3789, -80.428) -> (-127.3789, -76.428)
  arc A41 (-124.3789, -73.428) -> (-127.3789, -76.428) centre (-124.3789, -76.428) ccw
  line L42 (-124.3789, -73.428) -> (-120.3789, -73.428)
  arc A42 (-117.3789, -76.428) -> (-120.3789, -73.428) centre (-120.3789, -76.428) ccw
  line L43 (-117.3789, -76.428) -> (-117.3789, -80.428)
  arc A43 (-120.3789, -83.428) -> (-117.3789, -80.428) centre (-120.3789, -80.428) ccw
  line L44 (-149.6011, -68.8169) -> (-153.6011, -68.8169)
  arc A44 (-156.6011, -65.8169) -> (-153.6011, -68.8169) centre (-153.6011, -65.8169) ccw
  line L45 (-156.6011, -65.8169) -> (-156.6011, -61.8169)
  arc A45 (-153.6011, -58.8169) -> (-156.6011, -61.8169) centre (-153.6011, -61.8169) ccw
  line L46 (-153.6011, -58.8169) -> (-149.6011, -58.8169)
  arc A46 (-146.6011, -61.8169) -> (-149.6011, -58.8169) centre (-149.6011, -61.8169) ccw
  line L47 (-146.6011, -61.8169) -> (-146.6011, -65.8169)
  arc A47 (-149.6011, -68.8169) -> (-146.6011, -65.8169) centre (-149.6011, -65.8169) ccw
  line L48 (-76.5456, -171.0946) -> (-80.5456, -171.0946)
  arc A48 (-83.5456, -168.0946) -> (-80.5456, -171.0946) centre (-80.5456, -168.0946) ccw
  line L49 (-83.5456, -168.0946) -> (-83.5456, -164.0946)
  arc A49 (-80.5456, -161.0946) -> (-83.5456, -164.0946) centre (-80.5456, -164.0946) ccw
  line L50 (-80.5456, -161.0946) -> (-76.5456, -161.0946)
  arc A50 (-73.5456, -164.0946) -> (-76.5456, -161.0946) centre (-76.5456, -164.0946) ccw
  line L51 (-73.5456, -164.0946) -> (-73.5456, -168.0946)
  arc A51 (-76.5456, -171.0946) -> (-73.5456, -168.0946) centre (-76.5456, -168.0946) ccw
  line L52 (-105.7678, -68.8169) -> (-109.7678, -68.8169)
  arc A52 (-112.7678, -65.8169) -> (-109.7678, -68.8169) centre (-109.7678, -65.8169) ccw
  line L53 (-112.7678, -65.8169) -> (-112.7678, -61.8169)
  arc A53 (-109.7678, -58.8169) -> (-112.7678, -61.8169) centre (-109.7678, -61.8169) ccw
  line L54 (-109.7678, -58.8169) -> (-105.7678, -58.8169)
  arc A54 (-102.7678, -61.8169) -> (-105.7678, -58.8169) centre (-105.7678, -61.8169) ccw
  line L55 (-102.7678, -61.8169) -> (-102.7678, -65.8169)
  arc A55 (-105.7678, -68.8169) -> (-102.7678, -65.8169) centre (-105.7678, -65.8169) ccw
  line L56 (-120.3789, -171.0946) -> (-124.3789, -171.0946)
  arc A56 (-127.3789, -168.0946) -> (-124.3789, -171.0946) centre (-124.3789, -168.0946) ccw
  line L57 (-127.3789, -168.0946) -> (-127.3789, -164.0946)
  arc A57 (-124.3789, -161.0946) -> (-127.3789, -164.0946) centre (-124.3789, -164.0946) ccw
  line L58 (-124.3789, -161.0946) -> (-120.3789, -161.0946)
  arc A58 (-117.3789, -164.0946) -> (-120.3789, -161.0946) centre (-120.3789, -164.0946) ccw
  line L59 (-117.3789, -164.0946) -> (-117.3789, -168.0946)
  arc A59 (-120.3789, -171.0946) -> (-117.3789, -168.0946) centre (-120.3789, -168.0946) ccw
  line L60 (-134.99, -171.0946) -> (-138.99, -171.0946)
  arc A60 (-141.99, -168.0946) -> (-138.99, -171.0946) centre (-138.99, -168.0946) ccw
  line L61 (-141.99, -168.0946) -> (-141.99, -164.0946)
  arc A61 (-138.99, -161.0946) -> (-141.99, -164.0946) centre (-138.99, -164.0946) ccw
  line L62 (-138.99, -161.0946) -> (-134.99, -161.0946)
  arc A62 (-131.99, -164.0946) -> (-134.99, -161.0946) centre (-134.99, -164.0946) ccw
  line L63 (-131.99, -164.0946) -> (-131.99, -168.0946)
  arc A63 (-134.99, -171.0946) -> (-131.99, -168.0946) centre (-134.99, -168.0946) ccw
  line L64 (-164.2123, -156.4835) -> (-168.2123, -156.4835)
  arc A64 (-171.2123, -153.4835) -> (-168.2123, -156.4835) centre (-168.2123, -153.4835) ccw
  line L65 (-171.2123, -153.4835) -> (-171.2123, -149.4835)
  arc A65 (-168.2123, -146.4835) -> (-171.2123, -149.4835) centre (-168.2123, -149.4835) ccw
  line L66 (-168.2123, -146.4835) -> (-164.2123, -146.4835)
  arc A66 (-161.2123, -149.4835) -> (-164.2123, -146.4835) centre (-164.2123, -149.4835) ccw
  line L67 (-161.2123, -149.4835) -> (-161.2123, -153.4835)
  arc A67 (-164.2123, -156.4835) -> (-161.2123, -153.4835) centre (-164.2123, -153.4835) ccw
  line L68 (-32.7123, -112.6502) -> (-36.7123, -112.6502)
  arc A68 (-39.7123, -109.6502) -> (-36.7123, -112.6502) centre (-36.7123, -109.6502) ccw
  line L69 (-39.7123, -109.6502) -> (-39.7123, -105.6502)
  arc A69 (-36.7123, -102.6502) -> (-39.7123, -105.6502) centre (-36.7123, -105.6502) ccw
  line L70 (-36.7123, -102.6502) -> (-32.7123, -102.6502)
  arc A70 (-29.7123, -105.6502) -> (-32.7123, -102.6502) centre (-32.7123, -105.6502) ccw
  line L71 (-29.7123, -105.6502) -> (-29.7123, -109.6502)
  arc A71 (-32.7123, -112.6502) -> (-29.7123, -109.6502) centre (-32.7123, -109.6502) ccw
  line L72 (-76.5456, -68.8169) -> (-80.5456, -68.8169)
  arc A72 (-83.5456, -65.8169) -> (-80.5456, -68.8169) centre (-80.5456, -65.8169) ccw
  line L73 (-83.5456, -65.8169) -> (-83.5456, -61.8169)
  arc A73 (-80.5456, -58.8169) -> (-83.5456, -61.8169) centre (-80.5456, -61.8169) ccw
  line L74 (-80.5456, -58.8169) -> (-76.5456, -58.8169)
  arc A74 (-73.5456, -61.8169) -> (-76.5456, -58.8169) centre (-76.5456, -61.8169) ccw
  line L75 (-73.5456, -61.8169) -> (-73.5456, -65.8169)
  arc A75 (-76.5456, -68.8169) -> (-73.5456, -65.8169) centre (-76.5456, -65.8169) ccw
  line L76 (-61.9345, -68.8169) -> (-65.9345, -68.8169)
  arc A76 (-68.9345, -65.8169) -> (-65.9345, -68.8169) centre (-65.9345, -65.8169) ccw
  line L77 (-68.9345, -65.8169) -> (-68.9345, -61.8169)
  arc A77 (-65.9345, -58.8169) -> (-68.9345, -61.8169) centre (-65.9345, -61.8169) ccw
  line L78 (-65.9345, -58.8169) -> (-61.9345, -58.8169)
  arc A78 (-58.9345, -61.8169) -> (-61.9345, -58.8169) centre (-61.9345, -61.8169) ccw
  line L79 (-58.9345, -61.8169) -> (-58.9345, -65.8169)
  arc A79 (-61.9345, -68.8169) -> (-58.9345, -65.8169) centre (-61.9345, -65.8169) ccw
  line L80 (-91.1567, -54.2058) -> (-95.1567, -54.2058)
  arc A80 (-98.1567, -51.2058) -> (-95.1567, -54.2058) centre (-95.1567, -51.2058) ccw
  line L81 (-98.1567, -51.2058) -> (-98.1567, -47.2058)
  arc A81 (-95.1567, -44.2058) -> (-98.1567, -47.2058) centre (-95.1567, -47.2058) ccw
  line L82 (-95.1567, -44.2058) -> (-91.1567, -44.2058)
  arc A82 (-88.1567, -47.2058) -> (-91.1567, -44.2058) centre (-91.1567, -47.2058) ccw
  line L83 (-88.1567, -47.2058) -> (-88.1567, -51.2058)
  arc A83 (-91.1567, -54.2058) -> (-88.1567, -51.2058) centre (-91.1567, -51.2058) ccw
  line L84 (-76.5456, -39.5946) -> (-80.5456, -39.5946)
  arc A84 (-83.5456, -36.5946) -> (-80.5456, -39.5946) centre (-80.5456, -36.5946) ccw
  line L85 (-83.5456, -36.5946) -> (-83.5456, -32.5946)
  arc A85 (-80.5456, -29.5946) -> (-83.5456, -32.5946) centre (-80.5456, -32.5946) ccw
  line L86 (-80.5456, -29.5946) -> (-76.5456, -29.5946)
  arc A86 (-73.5456, -32.5946) -> (-76.5456, -29.5946) centre (-76.5456, -32.5946) ccw
  line L87 (-73.5456, -32.5946) -> (-73.5456, -36.5946)
  arc A87 (-76.5456, -39.5946) -> (-73.5456, -36.5946) centre (-76.5456, -36.5946) ccw
  line L88 (-47.3234, -98.0391) -> (-51.3234, -98.0391)
  arc A88 (-54.3234, -95.0391) -> (-51.3234, -98.0391) centre (-51.3234, -95.0391) ccw
  line L89 (-54.3234, -95.0391) -> (-54.3234, -91.0391)
  arc A89 (-51.3234, -88.0391) -> (-54.3234, -91.0391) centre (-51.3234, -91.0391) ccw
  line L90 (-51.3234, -88.0391) -> (-47.3234, -88.0391)
  arc A90 (-44.3234, -91.0391) -> (-47.3234, -88.0391) centre (-47.3234, -91.0391) ccw
  line L91 (-44.3234, -91.0391) -> (-44.3234, -95.0391)
  arc A91 (-47.3234, -98.0391) -> (-44.3234, -95.0391) centre (-47.3234, -95.0391) ccw
  line L92 (-47.3234, -83.428) -> (-51.3234, -83.428)
  arc A92 (-54.3234, -80.428) -> (-51.3234, -83.428) centre (-51.3234, -80.428) ccw
  line L93 (-54.3234, -80.428) -> (-54.3234, -76.428)
  arc A93 (-51.3234, -73.428) -> (-54.3234, -76.428) centre (-51.3234, -76.428) ccw
  line L94 (-51.3234, -73.428) -> (-47.3234, -73.428)
  arc A94 (-44.3234, -76.428) -> (-47.3234, -73.428) centre (-47.3234, -76.428) ccw
  line L95 (-44.3234, -76.428) -> (-44.3234, -80.428)
  arc A95 (-47.3234, -83.428) -> (-44.3234, -80.428) centre (-47.3234, -80.428) ccw
  line L96 (-47.3234, -112.6502) -> (-51.3234, -112.6502)
  arc A96 (-54.3234, -109.6502) -> (-51.3234, -112.6502) centre (-51.3234, -109.6502) ccw
  line L97 (-54.3234, -109.6502) -> (-54.3234, -105.6502)
  arc A97 (-51.3234, -102.6502) -> (-54.3234, -105.6502) centre (-51.3234, -105.6502) ccw
  line L98 (-51.3234, -102.6502) -> (-47.3234, -102.6502)
  arc A98 (-44.3234, -105.6502) -> (-47.3234, -102.6502) centre (-47.3234, -105.6502) ccw
  line L99 (-44.3234, -105.6502) -> (-44.3234, -109.6502)
  arc A99 (-47.3234, -112.6502) -> (-44.3234, -109.6502) centre (-47.3234, -109.6502) ccw
  line L100 (-76.5456, -112.6502) -> (-80.5456, -112.6502)
  arc A100 (-83.5456, -109.6502) -> (-80.5456, -112.6502) centre (-80.5456, -109.6502) ccw
  line L101 (-83.5456, -109.6502) -> (-83.5456, -105.6502)
  arc A101 (-80.5456, -102.6502) -> (-83.5456, -105.6502) centre (-80.5456, -105.6502) ccw
  line L102 (-80.5456, -102.6502) -> (-76.5456, -102.6502)
  arc A102 (-73.5456, -105.6502) -> (-76.5456, -102.6502) centre (-76.5456, -105.6502) ccw
  line L103 (-73.5456, -105.6502) -> (-73.5456, -109.6502)
  arc A103 (-76.5456, -112.6502) -> (-73.5456, -109.6502) centre (-76.5456, -109.6502) ccw
  line L104 (-32.7123, -83.428) -> (-36.7123, -83.428)
  arc A104 (-39.7123, -80.428) -> (-36.7123, -83.428) centre (-36.7123, -80.428) ccw
  line L105 (-39.7123, -80.428) -> (-39.7123, -76.428)
  arc A105 (-36.7123, -73.428) -> (-39.7123, -76.428) centre (-36.7123, -76.428) ccw
  line L106 (-36.7123, -73.428) -> (-32.7123, -73.428)
  arc A106 (-29.7123, -76.428) -> (-32.7123, -73.428) centre (-32.7123, -76.428) ccw
  line L107 (-29.7123, -76.428) -> (-29.7123, -80.428)
  arc A107 (-32.7123, -83.428) -> (-29.7123, -80.428) centre (-32.7123, -80.428) ccw
  line L108 (-91.1567, -98.0391) -> (-95.1567, -98.0391)
  arc A108 (-98.1567, -95.0391) -> (-95.1567, -98.0391) centre (-95.1567, -95.0391) ccw
  line L109 (-98.1567, -95.0391) -> (-98.1567, -91.0391)
  arc A109 (-95.1567, -88.0391) -> (-98.1567, -91.0391) centre (-95.1567, -91.0391) ccw
  line L110 (-95.1567, -88.0391) -> (-91.1567, -88.0391)
  arc A110 (-88.1567, -91.0391) -> (-91.1567, -88.0391) centre (-91.1567, -91.0391) ccw
  line L111 (-88.1567, -91.0391) -> (-88.1567, -95.0391)
  arc A111 (-91.1567, -98.0391) -> (-88.1567, -95.0391) centre (-91.1567, -95.0391) ccw
  line L112 (-47.3234, -39.5946) -> (-51.3234, -39.5946)
  arc A112 (-54.3234, -36.5946) -> (-51.3234, -39.5946) centre (-51.3234, -36.5946) ccw
  line L113 (-54.3234, -36.5946) -> (-54.3234, -32.5946)
  arc A113 (-51.3234, -29.5946) -> (-54.3234, -32.5946) centre (-51.3234, -32.5946) ccw
  line L114 (-51.3234, -29.5946) -> (-47.3234, -29.5946)
  arc A114 (-44.3234, -32.5946) -> (-47.3234, -29.5946) centre (-47.3234, -32.5946) ccw
  line L115 (-44.3234, -32.5946) -> (-44.3234, -36.5946)
  arc A115 (-47.3234, -39.5946) -> (-44.3234, -36.5946) centre (-47.3234, -36.5946) ccw
  line L116 (-76.5456, -54.2058) -> (-80.5456, -54.2058)
  arc A116 (-83.5456, -51.2058) -> (-80.5456, -54.2058) centre (-80.5456, -51.2058) ccw
  line L117 (-83.5456, -51.2058) -> (-83.5456, -47.2058)
  arc A117 (-80.5456, -44.2058) -> (-83.5456, -47.2058) centre (-80.5456, -47.2058) ccw
  line L118 (-80.5456, -44.2058) -> (-76.5456, -44.2058)
  arc A118 (-73.5456, -47.2058) -> (-76.5456, -44.2058) centre (-76.5456, -47.2058) ccw
  line L119 (-73.5456, -47.2058) -> (-73.5456, -51.2058)
  arc A119 (-76.5456, -54.2058) -> (-73.5456, -51.2058) centre (-76.5456, -51.2058) ccw
  line L120 (-76.5456, -83.428) -> (-80.5456, -83.428)
  arc A120 (-83.5456, -80.428) -> (-80.5456, -83.428) centre (-80.5456, -80.428) ccw
  line L121 (-83.5456, -80.428) -> (-83.5456, -76.428)
  arc A121 (-80.5456, -73.428) -> (-83.5456, -76.428) centre (-80.5456, -76.428) ccw
  line L122 (-80.5456, -73.428) -> (-76.5456, -73.428)
  arc A122 (-73.5456, -76.428) -> (-76.5456, -73.428) centre (-76.5456, -76.428) ccw
  line L123 (-73.5456, -76.428) -> (-73.5456, -80.428)
  arc A123 (-76.5456, -83.428) -> (-73.5456, -80.428) centre (-76.5456, -80.428) ccw
  line L124 (-91.1567, -68.8169) -> (-95.1567, -68.8169)
  arc A124 (-98.1567, -65.8169) -> (-95.1567, -68.8169) centre (-95.1567, -65.8169) ccw
  line L125 (-98.1567, -65.8169) -> (-98.1567, -61.8169)
  arc A125 (-95.1567, -58.8169) -> (-98.1567, -61.8169) centre (-95.1567, -61.8169) ccw
  line L126 (-95.1567, -58.8169) -> (-91.1567, -58.8169)
  arc A126 (-88.1567, -61.8169) -> (-91.1567, -58.8169) centre (-91.1567, -61.8169) ccw
  line L127 (-88.1567, -61.8169) -> (-88.1567, -65.8169)